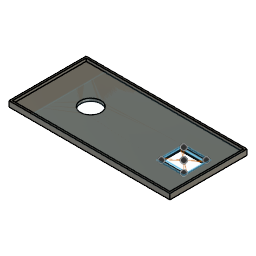
catlitter Top (Autodesk Fusion 360 design; units mm, degrees)
part number: 2025-12-03-17-21-50-791
Autodesk Fusion 360 part; units mm, degrees
sketch "Sketch1" plane through (0, 0, 0) normal (0, 0, 1) x (1, 0, 0)
  line L0 (76.5, 41.5) -> (-76.5, 41.5)
  line L1 (-76.5, 41.5) -> (-76.5, -41.5)
  line L2 (-76.5, -41.5) -> (76.5, -41.5)
  line L3 (76.5, -41.5) -> (76.5, 41.5)
  line L4 (76.5, 41.5) -> (-76.5, -41.5) construction
  line L5 (-76.5, 41.5) -> (76.5, -41.5) construction
  dimension "d1" = 153
  dimension "d2" = 83
  constraint horizontal L0
  constraint perpendicular L0 L1
  constraint parallel L0 L2
  constraint parallel L1 L3
  constraint coincident L4 origin
  constraint coincident L5 origin
  measures "d1" distance of L1.end L2.end
  measures "d2" distance of L0.end L1.end
extrude "Extrude1" add sketch "Sketch1" along normal blind 3
sketch "Sketch2" plane through (0, 0, 3) normal (0, 0, 1) x (-1, 0, 0)
  line L0 (-76.5, 41.5) -> (-76.5, -41.5)
  line L1 (-76.5, -41.5) -> (76.5, -41.5)
  line L2 (76.5, -41.5) -> (76.5, 41.5)
  line L3 (76.5, 41.5) -> (-76.5, 41.5)
  line L4 (-74.6, -39.6) -> (74.6, -39.6)
  line L5 (74.6, -39.6) -> (74.6, 39.6)
  line L6 (74.6, 39.6) -> (-74.6, 39.6)
  line L7 (-74.6, 39.6) -> (-74.6, -39.6)
  dimension "d5" = -1.9
extrude "Extrude2" add sketch "Sketch2" along normal blind 3
sketch "Sketch3" plane through (-76.5, 0, 0) normal (-1, 0, 0) x (0, -1, 0)
  line L0 (-41.5, 0) -> (41.5, 0)
  line L1 (41.5, 0) -> (41.5, 6)
  line L2 (41.5, 6) -> (-41.5, 6)
  line L3 (-41.5, 6) -> (-41.5, 0)
sketch "Sketch4" plane through (0, 0, 0) normal (0, 1, 0) x (1, 0, 0)
sketch "Sketch5" plane through (0, 0, 3) normal (0, 0, 1) x (-1, 0, 0)
  line L0 (-74.6, -39.6) -> (74.6, -39.6)
  line L1 (74.6, -39.6) -> (74.6, 39.6)
  line L2 (74.6, 39.6) -> (-74.6, 39.6)
  line L3 (-74.6, 39.6) -> (-74.6, -39.6)
  line L4 (-36.5, 10) -> (-63.5, 10)
  line L5 (-63.5, 10) -> (-63.5, -10)
  line L6 (-63.5, -10) -> (-36.5, -10)
  line L7 (-36.5, -10) -> (-36.5, 10)
  line L8 (-36.5, 10) -> (-63.5, -10) construction
  line L9 (-63.5, 10) -> (-36.5, -10) construction
  line L10 (-36, -14) -> (-64, -14)
  line L11 (-64, -14) -> (-64, 14)
  line L12 (-64, 14) -> (-36, 14)
  line L13 (-36, 14) -> (-36, -14)
  line L14 (-36, -14) -> (-64, 14) construction
  line L15 (-64, -14) -> (-36, 14) construction
  circle A0 centre (-37.9567, 12.0433) radius 1.5
  circle A1 centre (-61.9549, 11.9549) radius 1.5
  circle A2 centre (-62.1598, -12.1598) radius 1.5
  circle A3 centre (-37.9351, -12.0649) radius 1.5
  point P0 (-50, 0)
  point P1 (-50, 0)
  dimension "d8" = 27
  dimension "d9" = 20
  dimension "d12" = 28
  dimension "d13" = 28
  dimension "d14" = 3
  dimension "d15" = 3
  dimension "d16" = 3
  dimension "d17" = 3
  constraint horizontal L4
  constraint perpendicular L4 L5
  constraint parallel L4 L6
  constraint parallel L5 L7
  constraint coincident L8 P1
  constraint coincident L9 P1
  constraint horizontal L10
  constraint perpendicular L10 L11
  constraint parallel L10 L12
  constraint parallel L11 L13
  constraint coincident L14 P1
  constraint coincident L15 P1
  constraint coincident P1 P0
  constraint coincident L15 A0.centre
  constraint coincident L14 A1.centre
  constraint coincident L15 A2.centre
  constraint coincident L14 A3.centre
  measures "d8" distance of L5.end L6.end
  measures "d9" distance of L4.end L5.end
  measures "d12" distance of L11.end L12.end
  measures "d13" distance of L10.end L11.end
  measures "d14" diameter of A0
  measures "d15" diameter of A1
  measures "d16" diameter of A2
  measures "d17" diameter of A3
extrude "Extrude3" cut sketch "Sketch5" against normal blind 3 contours L4 L5 L6 L7
extrude "Extrude4" cut sketch "Sketch5" against normal blind 4 contours A0
extrude "Extrude5" cut sketch "Sketch5" against normal blind 4 contours A1
extrude "Extrude6" cut sketch "Sketch5" against normal blind 4 contours A2
extrude "Extrude7" cut sketch "Sketch5" against normal blind 5 contours A3
extrude "Extrude8" cut sketch "Sketch5" against normal blind 1.8 contours L10 L11 L12 L13
extrude "Extrude9" add sketch "Sketch3" along normal blind 20
move_face "OffsetFaces1" offset -20 1 faces at (-74.6, 13.2, 5)
sketch "Sketch6" plane through (0, 0, 3) normal (0, 0, 1) x (-1, 0, 0)
  circle A0 centre (50, 0) radius 11
  dimension "d31" = 22
  measures "d31" diameter of A0
extrude "Extrude10" cut sketch "Sketch6" against normal blind 5
